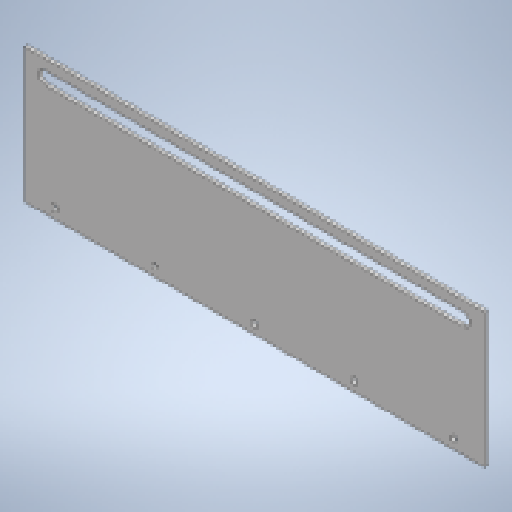
# Autodesk Inventor part: sokumen
Saved by Autodesk Inventor 2024 (Build 280153000, 153)
## iProperties
Created: 2024-06-08
Part Number: sokumen
Material: 一般
Document SubType Name: Modeling
Designer: right
Density: 1 g/cm^3
Appearance: 既定
Author: right
Autodesk Inventor part; units mm, degrees
ref_plane "YZ Plane" through (0, 0, 0) normal (1, 0, 0) x (0, 1, 0)
ref_plane "XZ Plane" through (0, 0, 0) normal (0, 1, 0) x (-1, 0, 0)
ref_plane "XY Plane" through (0, 0, 0) normal (0, 0, 1) x (1, 0, 0)
sketch "スケッチ1" plane through (0, 0, 0) normal (0, 0, 1) x (1, 0, 0)
  line L0 (52.5, 4.5) -> (252.5, 4.5) projected
  line L1 (252.5, 4.5) -> (252.5, 13.5) projected
  line L2 (252.5, 13.5) -> (250.93, 13.5) projected
  line L3 (250.93, 13.5) -> (247.786, 22.5) projected
  line L4 (247.786, 22.5) -> (244.6476, 22.5) projected
  line L5 (244.6476, 22.5) -> (241.5036, 13.5) projected
  line L6 (241.5036, 13.5) -> (238.3636, 13.5) projected
  line L7 (238.3636, 13.5) -> (235.2196, 22.5) projected
  line L8 (235.2196, 22.5) -> (232.0813, 22.5) projected
  line L9 (232.0813, 22.5) -> (228.9373, 13.5) projected
  line L10 (228.9373, 13.5) -> (225.7973, 13.5) projected
  line L11 (225.7973, 13.5) -> (222.6533, 22.5) projected
  line L12 (222.6533, 22.5) -> (219.5149, 22.5) projected
  line L13 (219.5149, 22.5) -> (216.3709, 13.5) projected
  line L14 (216.3709, 13.5) -> (213.2309, 13.5) projected
  line L15 (213.2309, 13.5) -> (210.0869, 22.5) projected
  line L16 (210.0869, 22.5) -> (206.9486, 22.5) projected
  line L17 (206.9486, 22.5) -> (203.8046, 13.5) projected
  line L18 (203.8046, 13.5) -> (200.6646, 13.5) projected
  line L19 (200.6646, 13.5) -> (197.5206, 22.5) projected
  line L20 (197.5206, 22.5) -> (194.3822, 22.5) projected
  line L21 (194.3822, 22.5) -> (191.2382, 13.5) projected
  line L22 (191.2382, 13.5) -> (188.0982, 13.5) projected
  line L23 (188.0982, 13.5) -> (184.9542, 22.5) projected
  line L24 (184.9542, 22.5) -> (181.8158, 22.5) projected
  line L25 (181.8158, 22.5) -> (178.6718, 13.5) projected
  line L26 (178.6718, 13.5) -> (175.5318, 13.5) projected
  line L27 (175.5318, 13.5) -> (172.3878, 22.5) projected
  line L28 (172.3878, 22.5) -> (169.2495, 22.5) projected
  line L29 (169.2495, 22.5) -> (166.1055, 13.5) projected
  line L30 (166.1055, 13.5) -> (162.9655, 13.5) projected
  line L31 (162.9655, 13.5) -> (159.8215, 22.5) projected
  line L32 (159.8215, 22.5) -> (156.6831, 22.5) projected
  line L33 (156.6831, 22.5) -> (153.5391, 13.5) projected
  line L34 (153.5391, 13.5) -> (150.3991, 13.5) projected
  line L35 (150.3991, 13.5) -> (147.2551, 22.5) projected
  line L36 (147.2551, 22.5) -> (144.1168, 22.5) projected
  line L37 (144.1168, 22.5) -> (140.9728, 13.5) projected
  line L38 (140.9728, 13.5) -> (137.8328, 13.5) projected
  line L39 (137.8328, 13.5) -> (134.6888, 22.5) projected
  line L40 (134.6888, 22.5) -> (131.5504, 22.5) projected
  line L41 (131.5504, 22.5) -> (128.4064, 13.5) projected
  line L42 (128.4064, 13.5) -> (125.2664, 13.5) projected
  line L43 (125.2664, 13.5) -> (122.1224, 22.5) projected
  line L44 (122.1224, 22.5) -> (118.984, 22.5) projected
  line L45 (118.984, 22.5) -> (115.84, 13.5) projected
  line L46 (115.84, 13.5) -> (112.7, 13.5) projected
  line L47 (112.7, 13.5) -> (109.556, 22.5) projected
  line L48 (109.556, 22.5) -> (106.4177, 22.5) projected
  line L49 (106.4177, 22.5) -> (103.2737, 13.5) projected
  line L50 (103.2737, 13.5) -> (100.1337, 13.5) projected
  line L51 (100.1337, 13.5) -> (96.9897, 22.5) projected
  line L52 (96.9897, 22.5) -> (93.8513, 22.5) projected
  line L53 (93.8513, 22.5) -> (90.7073, 13.5) projected
  line L54 (90.7073, 13.5) -> (87.5673, 13.5) projected
  line L55 (87.5673, 13.5) -> (84.4233, 22.5) projected
  line L56 (84.4233, 22.5) -> (81.285, 22.5) projected
  line L57 (81.285, 22.5) -> (78.141, 13.5) projected
  line L58 (78.141, 13.5) -> (75.001, 13.5) projected
  line L59 (75.001, 13.5) -> (71.857, 22.5) projected
  line L60 (71.857, 22.5) -> (68.7186, 22.5) projected
  line L61 (68.7186, 22.5) -> (65.5746, 13.5) projected
  line L62 (65.5746, 13.5) -> (62.4346, 13.5) projected
  line L63 (62.4346, 13.5) -> (59.2906, 22.5) projected
  line L64 (59.2906, 22.5) -> (56.1522, 22.5) projected
  line L65 (56.1522, 22.5) -> (53.0082, 13.5) projected
  line L66 (53.0082, 13.5) -> (52.5, 13.5) projected
  line L67 (52.5, 13.5) -> (52.5, 4.5) projected
  circle A0 centre (200.25, 9) radius 1.3 projected
  circle A1 centre (152.5, 9) radius 1.3 projected
  circle A2 centre (104.75, 9) radius 1.3 projected
  circle A3 centre (248, 9) radius 1.3 projected
  circle A4 centre (57, 9) radius 1.3 projected
  circle A5 centre (237.262, 60.7224) radius 6.2325 projected
  circle A6 centre (248, 9) radius 1.6
  circle A7 centre (200.25, 9) radius 1.6
  circle A8 centre (152.5, 9) radius 1.6
  circle A9 centre (104.75, 9) radius 1.6
  circle A10 centre (57, 9) radius 1.6
  circle A11 centre (237.262, 60.7224) radius 3
  circle A12 centre (52.5, 60.7224) radius 3
  line L68 (52.5, 57.7224) -> (252.5, 57.7224)
  line L69 (252.5, 57.7224) -> (252.5, 63.7224)
  line L70 (252.5, 63.7224) -> (52.5, 63.7224)
  line L71 (52.5, 63.7224) -> (52.5, 57.7224)
  circle A13 centre (252.5, 60.7224) radius 3
  line L72 (262.5, 4.5) -> (42.5, 4.5)
  line L73 (42.5, 4.5) -> (42.5, 111.8641)
  line L74 (42.5, 111.8641) -> (262.5, 111.8641)
  line L75 (262.5, 111.8641) -> (262.5, 4.5)
  arc A14 (214.0753, 100.6152) -> (211.159, 98.7709) centre (237.262, 60.7224) ccw projected
  circle A15 centre (237.262, 60.7224) radius 46.1417
  line L76 (237.262, 106.8641) -> (256.3928, 106.8641) construction
  circle A16 centre (224.125, 9) radius 1.3 projected
  circle A17 centre (80.875, 9) radius 1.3 projected
  circle A18 centre (176.375, 9) radius 1.3 projected
  circle A19 centre (128.625, 9) radius 1.3 projected
  point P0 (0, 0)
  point P1 (52.5, 63.7224)
  dimension "d6" = 6
  dimension "d0" = 3.2
  dimension "d1" = 3.2
  dimension "d2" = 3.2
  dimension "d3" = 3.2
  dimension "d4" = 3.2
  dimension "d5" = 6
  dimension "d8" = 10
  dimension "d9" = 10
  dimension "d12" = 5
  constraints: 18 end point, 7 centre point, 7 coincident, 5 horizontal, 4 parallel, 2 perpendicular, 2 point on circle, 2 vertical alignment, 1 horizontal alignment, 1 midpoint, 1 point on line, 1 tangent, 6 other
  measures "d0" diameter of A6
  measures "d1" diameter of A7
  measures "d2" diameter of A8
  measures "d3" diameter of A9
  measures "d4" diameter of A10
  measures "d5" diameter of A11
  measures "d8" distance from line of point (52.5, 60.722) L73
  measures "d9" distance from line of L75 L68.end
  measures "d12" distance between parallel lines of L74 L76
extrude "押し出し1" add sketch "スケッチ1" along normal blind 1.5 contours L67 L66 L65 L64 L63 L62 L61 L60 L59 L58 L57 L56 L55 L54 L53 L52 L51 L50 L49 L48 L47 L46 L45 L44 L43 L42 L41 L40 L39 L38 L37 L36 L35 L34 L33 L32 L31 L30 L29 L28 L27 L26 L25 L24 L23 L22 L21 L20 L19 L18 L17 L16 L15 L14 L13 A15 L11 L10 L9 L7 L6 L5 L3 L2 L1 L0 | L72 L73 L74 L75 A15 A14 L70 A12 L68 L13 L14 L15 L16 L17 L18 L19 L20 L21 L22 L23 L24 L25 L26 L27 L28 L29 L30 L31 L32 L33 L34 L35 L36 L37 L38 L39 L40 L41 L42 L43 L44 L45 L46 L47 L48 L49 L50 L51 L52 L53 L54 L55 L56 L57 L58 L59 L60 L61 L62 L63 L64 L65 L66 L67 | L1 L2 L3 A15 L75 L72 | A15 L3 L4 L5 L7 L8 L9 L11 L12 L13 L68 A5 A13 L70 A14 L75 | A15 L5 L4 L3 | L5 L6 L7 A15 | A15 L9 L8 L7 | L9 L10 L11 A15 | A15 L13 L12 L11 | A5 L70 | L68 A5 | A16 | A17 | A18 | A19
sketch "スケッチ2" plane through (0, 0, 0) normal (0, 0, -1) x (-1, 0, 0)
  circle A0 centre (-45, 109.3641) radius 2.5 construction
  line L0 (-262.5, 111.8641) -> (-42.5, 111.8641) projected
  line L1 (-42.5, 111.8641) -> (-42.5, 4.5) projected
  line L2 (-45, 109.3641) -> (-260, 109.3641) construction
  circle A1 centre (-260, 109.3641) radius 2.5 construction
  line L3 (-262.5, 4.5) -> (-262.5, 111.8641) construction
  line L4 (-230, 110.8641) -> (-220, 110.8641)
  line L5 (-220, 110.8641) -> (-220, 107.8641)
  line L6 (-220, 107.8641) -> (-230, 107.8641)
  line L7 (-230, 107.8641) -> (-230, 110.8641)
  line L8 (-230, 110.8641) -> (-220, 107.8641) construction
  line L9 (-220, 110.8641) -> (-230, 107.8641) construction
  circle A2 centre (-229.6, 108.2641) radius 1.1
  line L10 (-229.6, 108.2641) -> (-230, 107.8641) construction
  circle A3 centre (-229.6, 110.4641) radius 1.1
  line L11 (-225, 110.8641) -> (-225, 109.3641) construction
  line L12 (-220, 107.8641) -> (-220, 110.8641)
  circle A4 centre (-220.4, 108.2641) radius 1.1
  line L13 (-220.4, 108.2641) -> (-220, 107.8641) construction
  circle A5 centre (-220.4, 110.4641) radius 1.1
  circle A6 centre (-240, 109.3641) radius 1.1
  circle A7 centre (-210, 109.3641) radius 1.1
  line L14 (-152.5, 109.3641) -> (-152.5, 111.8641) construction
  line L15 (-75, 110.8641) -> (-85, 110.8641)
  line L16 (-85, 110.8641) -> (-85, 107.8641)
  line L17 (-85, 107.8641) -> (-75, 107.8641)
  line L18 (-75, 107.8641) -> (-75, 110.8641)
  line L19 (-75, 110.8641) -> (-85, 107.8641) construction
  line L20 (-85, 110.8641) -> (-75, 107.8641) construction
  circle A8 centre (-75.4, 108.2641) radius 1.1
  line L21 (-75.4, 108.2641) -> (-75, 107.8641) construction
  circle A9 centre (-75.4, 110.4641) radius 1.1
  line L22 (-80, 110.8641) -> (-80, 109.3641) construction
  line L23 (-84.6, 108.2641) -> (-85, 107.8641) construction
  line L24 (-85, 107.8641) -> (-85, 110.8641)
  circle A10 centre (-84.6, 108.2641) radius 1.1
  circle A11 centre (-84.6, 110.4641) radius 1.1
  circle A12 centre (-65, 109.3641) radius 1.1
  circle A13 centre (-95, 109.3641) radius 1.1
  point P0 (0, 0)
  point P1 (-85, 109.2888)
  point P2 (-83.5753, 107.8641)
  point P3 (-76.4247, 107.8641)
  point P4 (-75, 109.2888)
  point P5 (-75, 109.4394)
  point P6 (-76.4247, 110.8641)
  point P7 (-83.5753, 110.8641)
  point P8 (-85, 109.4394)
  point P9 (-221.4247, 110.8641)
  point P10 (-228.5753, 110.8641)
  point P11 (-230, 109.4394)
  point P12 (-230, 109.2888)
  point P13 (-228.5753, 107.8641)
  point P14 (-221.4247, 107.8641)
  point P15 (-220, 109.2888)
  point P16 (-220, 109.4394)
  dimension "d13" = 5
  dimension "d14" = 10
  dimension "d15" = 3
  dimension "d16" = 2.2
  dimension "d17" = 45
  dimension "d18" = 2.2
  dimension "d19" = 10
  dimension "d20" = 20
  constraints: 44 end point, 16 symmetric about line, 14 centre point, 5 midpoint, 5 tangent, 3 parallel, 2 point on line, 1 coincident, 1 horizontal, 1 perpendicular, 10 other
  measures "d13" diameter of A0
  measures "d14" distance of L5.end L6.end
  measures "d15" distance of L4.end L5.end
  measures "d16" diameter of A2
  measures "d17" angle of L7 L10
  measures "d18" diameter of A6
  measures "d19" distance from line of L7 A6.centre
  measures "d20" distance of L2.end A6.centre
extrude "押し出し2" cut sketch "スケッチ2" against normal through all
sketch "スケッチ3" plane through (0, 0, 1.5) normal (0, 0, 1) x (1, 0, 0)
  line L0 (32.5, 4.5) -> (32.5, 111.8641) projected
  line L1 (32.5, 111.8641) -> (272.5, 111.8641) projected
  line L2 (272.5, 4.5) -> (32.5, 4.5) projected
  line L3 (42.5, 111.8641) -> (42.5, 4.5) projected
  point P0 (0, 0)
extrude "押し出し3" add sketch "スケッチ3" against normal up to surface (1.5 mm away)
chamfer "面取り1" distance 23.25 angle 45 1 edges at (32.5, 4.5, 0.75)
sketch "スケッチ6" plane through (0, 0, 1.5) normal (0, 0, 1) x (1, 0, 0)
  circle A0 centre (44.5, 12.5) radius 8 projected
  line L0 (32.5, 27.75) -> (32.5, 111.8641) projected
  line L1 (48.1883, 19.599) -> (32.5, 27.75)
  line L2 (55.75, 4.5) -> (32.5, 27.75) projected
  point P0 (0, 0)
  point P1 (51.5434, 8.7066)
  constraints: 2 end point, 3 other
extrude "押し出し6" cut sketch "スケッチ6" against normal through all contours A0 L2 | A0 L2 L1 picked at (48.9651, 14.7984)
fillet "フィレット2" radius 2 1 edges at (51.5434, 8.7066, 0.75)
equation "\"d9\" = d8"
